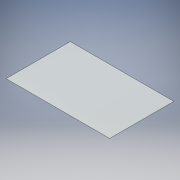
# Autodesk Inventor part: coffeeWindowSide
Saved by Autodesk Inventor 2019 (Build 230136000, 136)
## iProperties
Created: 2018-10-08
Part Number: coffeeWindowSide
Material: Glass
Document SubType Name: Modeling
Designer: wade
Density: 2.18 g/cm^3
Appearance: Clear
Author: wade
Autodesk Inventor part; units mm, degrees
ref_plane "YZ Plane" through (0, 0, 0) normal (1, 0, 0) x (0, 1, 0)
ref_plane "XZ Plane" through (0, 0, 0) normal (0, 1, 0) x (-1, 0, 0)
ref_plane "XY Plane" through (0, 0, 0) normal (0, 0, 1) x (1, 0, 0)
sketch "Sketch1" plane through (0, 0, 0) normal (0, 1, 0) x (-1, 0, 0)
  line L0 (0, 0) -> (5000, 0)
  line L1 (5000, 0) -> (5000, -3100)
  line L2 (5000, -3100) -> (0, -3100)
  line L3 (0, -3100) -> (0, 0)
  dimension "d0" = 5000
  dimension "d1" = 3100
  constraints: 8 end point, 2 parallel, 1 horizontal, 1 perpendicular
  measures "d0" distance of L1.end L2.end
  measures "d1" distance of L0.end L1.end
extrude "Extrusion1" add sketch "Sketch1" along normal blind 10
body "Solid1"
